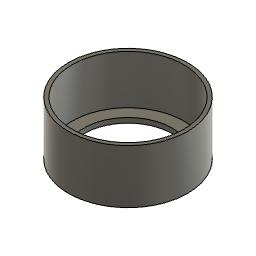
viewport_frame v2 (Autodesk Fusion 360 design; units mm, degrees)
Autodesk Fusion 360 part; units mm, degrees
sketch "Sketch1" plane through (0, 0, 0) normal (0, 1, 0) x (1, 0, 0)
  circle A0 centre (0, 0) radius 61
  dimension "d2" = 122
  measures "d2" diameter of A0
extrude "Extrude1" add sketch "Sketch1" along normal blind 5
sketch "Sketch3" plane through (0, 5, 0) normal (0, 1, 0) x (-1, 0, 0)
  circle A0 centre (0, 0) radius 61
  circle A1 centre (0, 0) radius 61
  circle A2 centre (0, 0) radius 57.25
  dimension "d5" = 114.5
  constraint coincident A0.centre A1.centre
  constraint concentric A1 A2
  measures "d5" diameter of A2
extrude "Extrude2" add sketch "Sketch3" along normal blind 50
sketch "Sketch4" plane through (0, 5, 0) normal (0, 1, 0) x (-1, 0, 0)
  circle A0 centre (0, 0) radius 57.25
  circle A1 centre (0, 0) radius 45
  dimension "d8" = 90
  constraint coincident A0.centre A1.centre
  measures "d8" diameter of A1
extrude "Extrude3" cut sketch "Sketch4" against normal blind 55 contours A1
